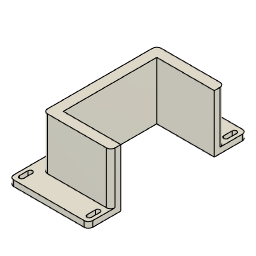
Battery+Mount (Autodesk Fusion 360 design; units mm, degrees)
Autodesk Fusion 360 part; units mm, degrees
sketch "Sketch1" plane through (0, 0, 0) normal (0, 1, 0) x (1, 0, 0)
  line L0 (0, 0) -> (55, 0)
  line L1 (0, 0) -> (0, 110)
  line L2 (0, 110) -> (55, 110)
  line L3 (55, 110) -> (55, 94.5)
  line L4 (55, 94.5) -> (8, 94.5)
  line L5 (8, 94.5) -> (8, 15.5)
  line L6 (8, 15.5) -> (55, 15.5)
  line L7 (55, 15.5) -> (55, 0)
  line L8 (55, 15.5) -> (55, 22.5)
  line L9 (55, 22.5) -> (15, 22.5)
  line L10 (15, 22.5) -> (15, 87.5)
  line L11 (15, 87.5) -> (55, 87.5)
  line L12 (55, 87.5) -> (55, 94.5)
  line L13 (4, 0) -> (4, 110) construction
  circle A0 centre (51, 7.5) radius 1.55
  circle A1 centre (4, 7.5) radius 1.55
  circle A2 centre (4, 102.5) radius 1.55
  circle A3 centre (51, 102.5) radius 1.55
  circle A4 centre (4, 70.84) radius 1.55
  circle A5 centre (4, 39.16) radius 1.55
  line L14 (52.55, 4.5) -> (52.55, 10.5)
  arc A6 (52.55, 10.5) -> (49.45, 10.5) centre (51, 10.5) ccw
  line L15 (49.45, 10.5) -> (49.45, 4.5)
  arc A7 (49.45, 4.5) -> (52.55, 4.5) centre (51, 4.5) ccw
  line L16 (51, 4.5) -> (51, 10.5) construction
  line L17 (51, 99.5) -> (51, 105.5) construction
  line L18 (5.55, 99.5) -> (5.55, 105.5)
  arc A8 (5.55, 105.5) -> (2.45, 105.5) centre (4, 105.5) ccw
  line L19 (2.45, 105.5) -> (2.45, 99.5)
  arc A9 (2.45, 99.5) -> (5.55, 99.5) centre (4, 99.5) ccw
  line L20 (4, 99.5) -> (4, 105.5) construction
  line L21 (52.55, 99.5) -> (52.55, 105.5)
  arc A10 (52.55, 105.5) -> (49.45, 105.5) centre (51, 105.5) ccw
  line L22 (49.45, 105.5) -> (49.45, 99.5)
  arc A11 (49.45, 99.5) -> (52.55, 99.5) centre (51, 99.5) ccw
  line L23 (51, 99.5) -> (51, 105.5) construction
  line L24 (5.55, 4.5) -> (5.55, 10.5)
  arc A12 (5.55, 10.5) -> (2.45, 10.5) centre (4, 10.5) ccw
  line L25 (2.45, 10.5) -> (2.45, 4.5)
  arc A13 (2.45, 4.5) -> (5.55, 4.5) centre (4, 4.5) ccw
  line L26 (4, 4.5) -> (4, 10.5) construction
  point P0 (51, 7.5)
  point P1 (51, 102.5)
  point P2 (4, 102.5)
  point P3 (51, 102.5)
  point P4 (4, 7.5)
  dimension "d1" = 65
  dimension "d2" = 7
  dimension "d3" = 15.5
  dimension "d4" = 7
  dimension "d5" = 8
  dimension "d7" = 40
  dimension "d8" = 4
  dimension "d9" = 3.1
  dimension "d10" = 3.1
  dimension "d11" = 3.1
  dimension "d12" = 3.1
  dimension "d14" = 4
  dimension "d15" = 4
  dimension "d34" = 7.5
  dimension "d35" = 7.5
  dimension "d36" = 7.5
  dimension "d37" = 7.5
  dimension "d38" = 3.1
  dimension "d39" = 3.1
  dimension "d40" = 31.66
  dimension "d41" = 31.66
  dimension "d42" = 3.1
  dimension "d43" = 3.1
  dimension "d44" = 3.1
  dimension "d45" = 3.1
  dimension "d46" = 3
  dimension "d47" = 3
  dimension "d48" = 3
  dimension "d49" = 3
  constraint coincident L0.start L1.start
  constraint horizontal L0
  constraint perpendicular L0 L1
  constraint perpendicular L1 L2
  constraint perpendicular L2 L3
  constraint perpendicular L3 L4
  constraint perpendicular L2 L5
  constraint perpendicular L5 L6
  constraint perpendicular L0 L7
  constraint perpendicular L6 L8
  constraint perpendicular L7 L9
  constraint perpendicular L6 L10
  constraint perpendicular L10 L11
  constraint perpendicular L4 L12
  constraint equal L9 L11
  constraint equal L8 L12
  constraint equal L3 L7
  constraint coincident L0 L13.start
  constraint coincident L2 L13.end
  constraint perpendicular L2 L13
  constraint coincident L13 P4
  constraint coincident L13 P2
  constraint coincident L13 A4.centre
  constraint coincident L13 A5.centre
  constraint tangent L14 A6
  constraint tangent A6 L15
  constraint parallel L14 L15
  constraint tangent L15 A7
  constraint tangent L14 A7
  constraint perpendicular L6 L16
  constraint coincident P0 A0.centre
  constraint midpoint L16 P0
  constraint vertical L17
  constraint coincident P3 P1
  constraint midpoint L17 P3
  constraint tangent L18 A8
  constraint tangent A8 L19
  constraint parallel L18 L19
  constraint tangent L19 A9
  constraint tangent L18 A9
  constraint parallel L13 L20
  constraint coincident P2 A2.centre
  constraint midpoint L20 P2
  constraint tangent L21 A10
  constraint tangent A10 L22
  constraint parallel L21 L22
  constraint tangent L22 A11
  constraint tangent L21 A11
  constraint parallel L17 L23
  constraint midpoint L23 P3
  constraint tangent L24 A12
  constraint tangent A12 L25
  constraint parallel L24 L25
  constraint tangent L25 A13
  constraint tangent L24 A13
  constraint parallel L13 L26
  constraint coincident P4 A1.centre
  constraint midpoint L26 P4
  constraint coincident L17.end A10.centre
  measures "d1" distance of L9 L11
  measures "d2" distance of L6.end L8.end
  measures "d3" distance of L0.end L6.end
  measures "d4" distance of L5 L10
  measures "d5" distance of L1 L5
  measures "d7" distance of L8.end L9.end
  measures "d8" distance of L1 L13
  measures "d9" diameter of A0
  measures "d10" diameter of A1
  measures "d11" diameter of A2
  measures "d12" diameter of A3
  measures "d14" distance of L7 P0
  measures "d15" distance of L3 P3
  measures "d34" distance of L2 P3
  measures "d35" distance of L2 P2
  measures "d36" distance of L0 P0
  measures "d37" distance of L0 P4
  measures "d38" diameter of A4
  measures "d39" diameter of A5
  measures "d40" distance of P2 A4.centre
  measures "d41" distance of P4 A5.centre
  measures "d42" diameter of A6
  measures "d43" diameter of A8
  measures "d44" diameter of A10
  measures "d45" diameter of A12
  measures "d46" distance of A8.centre P2
  measures "d47" distance of L17.end P3
  measures "d48" distance of P4 A12.centre
  measures "d49" distance of A6.centre P0
extrude "Extrude1" add sketch "Sketch1" along normal blind 4 contours L0 L1 L2 L3 L4 L5 L6 L7
extrude "Extrude2" add sketch "Sketch1" along normal blind 40 contours L4 L5 L6 L8 L9 L10 L11 L12
fillet "Fillet1" radius 3 6 edges at (55, 2, 0) (8, 22, -15.5) (0, 2, 0) (55, 2, -110) (8, 22, -94.5) (0, 2, -110)
fillet "Fillet1" radius 3 2 edges at (55, 22, -94.5) (55, 22, -15.5)
equation "d4 = d2"
equation "d10 = d9"
equation "d15 = d14"
equation "d42 = d9"
equation "d43 = d9"
equation "d44 = d9"
equation "d45 = d9"
equation "d47 = d46"
equation "d48 = d46"
equation "d49 = d46"
